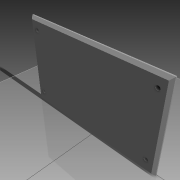
# Autodesk Inventor part: Enclosure-Backplate01
Saved by Autodesk Inventor 2013 (Build 170138000, 138)
## iProperties
Created: 2014-04-13
Part Number: Enclosure-Backplate01
Material: Generic
Document SubType Name: Modeling
Designer: spichelh
Density: 1 g/cm^3
Author: spichelh
Autodesk Inventor part; units mm, degrees
ref_plane "YZ Plane" through (0, 0, 0) normal (1, 0, 0) x (0, 1, 0)
ref_plane "XZ Plane" through (0, 0, 0) normal (0, 1, 0) x (-1, 0, 0)
ref_plane "XY Plane" through (0, 0, 0) normal (0, 0, 1) x (1, 0, 0)
sketch "Sketch1" plane through (0, 0, 0) normal (0, 0, 1) x (1, 0, 0)
  line L0 (-57.5279, 33.0143) -> (-57.5279, -34.9857) projected
  line L1 (50.0721, 33.0143) -> (24.2721, 33.0143) projected
  line L2 (50.0721, -34.9857) -> (50.0721, 33.0143) projected
  line L3 (-57.5279, -34.9857) -> (-31.7279, -34.9857) projected
  line L4 (-31.7279, 33.0143) -> (-57.5279, 33.0143) projected
  line L5 (50.0721, 33.0143) -> (-57.5279, 33.0143)
  line L6 (-57.5279, 33.0143) -> (-57.5279, -34.9857)
  line L7 (50.0721, -34.9857) -> (50.0721, 33.0143)
  line L8 (-31.6679, -34.9857) -> (24.2121, -34.9857) projected
  line L9 (24.2121, -34.9857) -> (24.2121, -29.9857) projected
  line L10 (24.2121, -29.9857) -> (-31.6679, -29.9857) projected
  line L11 (-31.6679, -29.9857) -> (-31.6679, -34.9857) projected
  line L12 (-57.5279, -34.9857) -> (50.0721, -34.9857)
  point P0 (50.3721, -34.9957)
  point P1 (50.3721, 48.8143)
  point P2 (-57.2279, -34.9957)
  dimension "d16" = 107.6
  dimension "d17" = 83.81
  constraints: 8 end point, 1 collinear, 1 horizontal, 1 parallel, 1 perpendicular
  measures "d16" distance of point (50.372, -34.996) point (-57.228, -34.996)
  measures "d17" distance of point (50.372, 48.814) point (50.372, -34.996)
extrude "Extrusion1" add sketch "Sketch1" along normal blind 3
sketch "Sketch2" plane through (0, 0, 0) normal (0, 0, -1) x (-1, 0, 0)
  line L0 (57.5279, -34.9857) -> (57.5279, 33.0143) projected
  line L1 (57.5279, 33.0143) -> (-50.0721, 33.0143) projected
  line L2 (-50.0721, 33.0143) -> (-50.0721, -34.9857) projected
  line L3 (54.9279, 30.4143) -> (-47.4721, 30.4143)
  line L4 (-47.4721, 30.4143) -> (-47.4721, -32.3857)
  line L5 (54.9279, -32.3857) -> (54.9279, 30.4143)
  line L6 (-50.0721, -34.9857) -> (57.5279, -34.9857) projected
  line L7 (31.6679, -34.9857) -> (-24.2121, -34.9857) projected
  line L8 (-24.2121, -34.9857) -> (-24.2121, -29.9857) projected
  line L9 (-24.2121, -29.9857) -> (31.6679, -29.9857) projected
  line L10 (31.6679, -29.9857) -> (31.6679, -34.9857) projected
  line L11 (-47.4721, -32.3857) -> (-24.2121, -32.3857)
  line L12 (31.6679, -32.3857) -> (54.9279, -32.3857)
  line L13 (31.6679, -32.3857) -> (31.6679, -29.9857)
  line L14 (-24.2121, -29.9857) -> (-24.2121, -32.3857)
  line L15 (31.6679, -29.9857) -> (-24.2121, -29.9857)
  dimension "d28" = 2.6
  dimension "d29" = 2.6
  dimension "d30" = 2.6
  constraints: 16 end point, 3 collinear, 3 parallel, 2 point on line, 1 horizontal, 1 perpendicular
  measures "d28" distance between parallel lines of L1 L3
  measures "d29" distance between parallel lines of L5 L0
  measures "d30" distance between parallel lines of L2 L4
extrude "Extrusion2" add sketch "Sketch2" along normal blind 1 contours L10 L9 L8 L11 L4 L3 L5 L12
sketch "Sketch3" plane through (0, 0, 3) normal (0, 0, 1) x (1, 0, 0)
  circle A0 centre (-50.7179, 24.5443) radius 1.5 projected
  circle A1 centre (-50.7179, -24.9857) radius 1.5 projected
  circle A2 centre (43.2621, -24.9857) radius 1.5 projected
  circle A3 centre (43.2621, 24.5443) radius 1.5 projected
  point P0 (0, 0)
extrude "Extrusion3" cut sketch "Sketch3" against normal blind 4
chamfer "Chamfer2" distance 2 angle 45 3 edges at (-3.7279, 33.0143, 3) (-57.5279, -0.9857, 3) (50.0721, -0.9857, 3)
body "Solid1"
